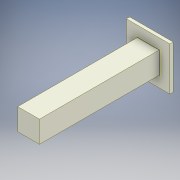
# Autodesk Inventor part: TagPillar
Saved by Autodesk Inventor 2018 (Build 220112000, 112)
## iProperties
Created: 2018-09-24
Part Number: TagPillar
Material: Generic
Document SubType Name: Modeling
Designer: DCCUMD
Density: 1 g/cm^3
Appearance: Smooth - Ivory
Author: DCCUMD
Autodesk Inventor part; units mm, degrees
ref_plane "YZ Plane" through (0, 0, 0) normal (1, 0, 0) x (0, 1, 0)
ref_plane "XZ Plane" through (0, 0, 0) normal (0, 1, 0) x (-1, 0, 0)
ref_plane "XY Plane" through (0, 0, 0) normal (0, 0, 1) x (1, 0, 0)
sketch "Sketch1" plane through (0, 0, 0) normal (0, 1, 0) x (-1, 0, 0)
  line L0 (0, 0) -> (20, 0)
  line L1 (20, 0) -> (20, -20)
  line L2 (20, -20) -> (0, -20)
  line L3 (0, -20) -> (0, 0)
  dimension "d0" = 20
  dimension "d1" = 20
  constraints: 8 end point, 2 parallel, 1 horizontal, 1 perpendicular
  measures "d0" distance of L1.end L2.end
  measures "d1" distance of L0.end L1.end
extrude "Extrusion1" add sketch "Sketch1" along normal blind 110
ref_plane "Work Plane1" through (-20, 110, -10) normal (0, 1, 0) x (1, 0, 0)
sketch "Sketch3" plane through (-20, 110, -10) normal (0, 1, 0) x (1, 0, 0)
  line L0 (0, -10) -> (20, -10) projected
  line L1 (20, -10) -> (20, 10) projected
  line L2 (30, -20) -> (-10, -20)
  line L3 (-10, -20) -> (-10, 20)
  line L4 (-10, 20) -> (30, 20)
  line L5 (30, 20) -> (30, -20)
  line L6 (30, -20) -> (-10, 20) construction
  line L7 (-10, -20) -> (30, 20) construction
  point P0 (10, 0)
  dimension "d4" = 10
  dimension "d5" = 10
  dimension "d6" = 40
  dimension "d7" = 40
  constraints: 12 end point, 2 midpoint, 2 parallel, 1 horizontal, 1 perpendicular
  measures "d4" distance from line of L0 point (10, 0)
  measures "d5" distance from line of L1 point (10, 0)
  measures "d6" distance of L3.end L4.end
  measures "d7" distance of L2.end L3.end
extrude "Extrusion2" add sketch "Sketch3" along normal blind 3
body "Solid1"
